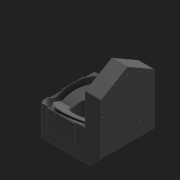
# Autodesk Inventor part: Arm L-Bracket
Saved by Autodesk Inventor 2017 (Build 210142000, 142)
## iProperties
Created: 2019-08-29
Part Number: Arm L-Bracket
Material: ABS Plastic
Document SubType Name: Modeling
Designer: Dell
Density: 1.06 g/cm^3
Appearance: Smooth - Black
Author: Dell
Autodesk Inventor part; units mm, degrees
ref_plane "YZ Plane" through (0, 0, 0) normal (1, 0, 0) x (0, 1, 0)
ref_plane "XZ Plane" through (0, 0, 0) normal (0, 1, 0) x (-1, 0, 0)
ref_plane "XY Plane" through (0, 0, 0) normal (0, 0, 1) x (1, 0, 0)
sketch "Sketch1" plane through (0, 0, 0) normal (0, 0, 1) x (1, 0, 0)
  line L0 (68.1273, 0) -> (34.0637, -59)
  line L1 (34.0637, -59) -> (-34.0637, -59)
  line L2 (-34.0637, -59) -> (-68.1273, 0)
  line L3 (-68.1273, 0) -> (-34.0637, 59)
  line L4 (-34.0637, 59) -> (34.0637, 59)
  line L5 (34.0637, 59) -> (68.1273, 0)
  line L6 (34.0637, 59) -> (43.0281, 59)
  line L7 (43.0281, 59) -> (93.1273, 59)
  line L8 (93.1273, 59) -> (93.1273, -59)
  line L9 (93.1273, -59) -> (34.0637, -59)
  circle A0 centre (0, 0) radius 22.5
  circle A1 centre (-54, 0) radius 2.5
  circle A2 centre (-46.7654, -27) radius 2.5
  circle A3 centre (-27, -46.7654) radius 2.5
  circle A4 centre (0, -54) radius 2.5
  circle A5 centre (27, -46.7654) radius 2.5
  circle A6 centre (46.7654, -27) radius 2.5
  circle A7 centre (54, 0) radius 2.5
  circle A8 centre (46.7654, 27) radius 2.5
  circle A9 centre (27, 46.7654) radius 2.5
  circle A10 centre (0, 54) radius 2.5
  circle A11 centre (-27, 46.7654) radius 2.5
  circle A12 centre (-46.7654, 27) radius 2.5
  dimension "d0" = 118
  dimension "d1" = 25
  dimension "d2" = 45
  dimension "d3" = 54
  dimension "d4" = 5
  dimension "d7" = 360
  constraints: 20 end point, 13 centre point, 2 coincident, 2 horizontal, 2 horizontal alignment, 1 perpendicular, 1 point on line, 38 other
  measures "d0" distance between parallel lines of L1 L4
  measures "d1" distance from line of L8 L0.start
  measures "d2" diameter of A0
  measures "d3" distance of point (0, 0) A1.centre
  measures "d4" diameter of A1
extrude "Extrusion1" add sketch "Sketch1" along normal blind 30
sketch "Sketch2" plane through (93.1273, -59, 0) normal (1, 0, 0) x (0, 0, -1)
  line L0 (-69.0637, 118) -> (-35, 59)
  line L1 (-35, 59) -> (-69.0637, 0)
  line L2 (-69.0637, 0) -> (-137.191, 0)
  line L3 (-137.191, 0) -> (-171.2547, 59)
  line L4 (-171.2547, 59) -> (-137.191, 118)
  line L5 (-137.191, 118) -> (-69.0637, 118)
  line L6 (0, 0) -> (0, 118) projected
  line L7 (0, 0) -> (-69.0637, 0)
  line L8 (0, 118) -> (-30, 118) projected
  line L9 (-69.0637, 118) -> (0, 118)
  line L10 (0, 118) -> (0, 0)
  circle A0 centre (-103.1273, 59) radius 22.5
  circle A1 centre (-157.1273, 59) radius 2.5
  circle A2 centre (-149.8927, 32) radius 2.5
  circle A3 centre (-130.1273, 12.2346) radius 2.5
  circle A4 centre (-103.1273, 5) radius 2.5
  circle A5 centre (-76.1273, 12.2346) radius 2.5
  circle A6 centre (-56.362, 32) radius 2.5
  circle A7 centre (-49.1273, 59) radius 2.5
  circle A8 centre (-56.362, 86) radius 2.5
  circle A9 centre (-76.1273, 105.7654) radius 2.5
  circle A10 centre (-103.1273, 113) radius 2.5
  circle A11 centre (-130.1273, 105.7654) radius 2.5
  circle A12 centre (-149.8927, 86) radius 2.5
  point P0 (0, 59)
  point P1 (-30, 0)
  dimension "d12" = 45
  dimension "d13" = 5
  dimension "d14" = 54
  dimension "d17" = 360
  dimension "d25" = 5
  constraints: 18 end point, 13 centre point, 3 horizontal alignment, 2 perpendicular, 1 coincident, 1 collinear, 1 horizontal, 38 other
  measures "d12" diameter of A0
  measures "d13" diameter of A1
  measures "d14" distance of point (-103.127, 59) A1.centre
  measures "d25" horizontal distance of L8.end L0.end
extrude "Extrusion2" add sketch "Sketch2" against normal blind 30 and the other way blind 5
sketch "Sketch3" plane through (63.1273, -59, 0) normal (-1, 0, 0) x (0, 0, 1)
  circle A0 centre (103.1273, 59) radius 22.5 projected
  line L0 (171.2547, 59) -> (137.191, 0) projected
  line L1 (171.2547, 59) -> (137.191, 0)
  line L2 (137.191, 0) -> (69.0637, 0)
  line L3 (69.0637, 0) -> (35, 59)
  line L4 (35, 59) -> (69.0637, 118)
  line L5 (69.0637, 118) -> (137.191, 118)
  line L6 (137.191, 118) -> (171.2547, 59)
  line L7 (137.191, 118) -> (30, 118) projected
  line L8 (69.0637, 118) -> (30, 118)
  line L9 (30, 0) -> (30, 118) projected
  line L10 (30, 118) -> (30, 0)
  line L11 (30, 0) -> (69.0637, 0)
  point P0 (0, 59)
  constraints: 18 end point, 2 collinear, 1 coincident, 1 perpendicular, 13 other
extrude "Extrusion3" add sketch "Sketch3" along normal blind 180 contours L11 L9 L7 L4 L3
sketch "Sketch4" plane through (0, 0, 0) normal (0, 0, -1) x (-1, 0, 0)
  line L0 (34.0637, -59) -> (-98.1273, -59) projected
  line L1 (68.1273, 0) -> (34.0637, -59) projected
  line L2 (34.0637, 59) -> (68.1273, 0) projected
  line L3 (34.0637, 59) -> (-98.1273, 59) projected
  line L4 (-98.1273, -59) -> (-98.1273, 59) construction
  circle A0 centre (0, 0) radius 22.5 projected
  circle A1 centre (46.7654, 27) radius 2.5 projected
  circle A2 centre (27, 46.7654) radius 2.5 projected
  circle A3 centre (0, 54) radius 2.5 projected
  circle A4 centre (-27, 46.7654) radius 2.5 projected
  circle A5 centre (-46.7654, 27) radius 2.5 projected
  circle A6 centre (-54, 0) radius 2.5 projected
  circle A7 centre (-46.7654, -27) radius 2.5 projected
  circle A8 centre (-27, -46.7654) radius 2.5 projected
  circle A9 centre (0, -54) radius 2.5 projected
  circle A10 centre (27, -46.7654) radius 2.5 projected
  circle A11 centre (46.7654, -27) radius 2.5 projected
  circle A12 centre (54, 0) radius 2.5 projected
  line L5 (34.0637, 59) -> (68.1273, 0) projected
  line L6 (68.1273, 0) -> (34.0637, -59) projected
  line L7 (34.0637, -59) -> (116.8727, -59) projected
  line L8 (116.8727, 59) -> (116.8727, -59) projected
  line L9 (34.0637, 59) -> (116.8727, 59) projected
extrude "Extrusion4" cut sketch "Sketch4" against normal through all
sketch "Sketch5" plane through (98.1273, -59, 0) normal (1, 0, 0) x (0, 0, -1)
  circle A0 centre (-103.1273, 59) radius 22.5 projected
extrude "Extrusion5" add sketch "Sketch5" against normal blind 5
sketch "Sketch6" plane through (63.1273, -59, 0) normal (-1, 0, 0) x (0, 0, 1)
  circle A0 centre (103.1273, 59) radius 22.5 projected
  line L0 (82.8587, 68.7691) -> (46.8217, 79.4757)
  line L1 (80.6273, 59) -> (41.6806, 70.5711)
  line L2 (69.0637, 118) -> (35, 59) projected
  line L3 (69.0637, 118) -> (35, 59) projected
  circle A1 centre (56.362, 86) radius 2.5 construction
  circle A2 centre (49.1273, 59) radius 2.5 construction
  circle A3 centre (56.362, 86) radius 2.5 projected
  line L4 (56.362, 86) -> (54.0392, 77.3314)
  line L5 (49.1273, 59) -> (51.4501, 67.6686)
  line L6 (54.0392, 77.3314) -> (51.4501, 67.6686) construction
  circle A4 centre (49.1273, 59) radius 2.5 projected
  line L7 (103.1273, 59) -> (49.1273, 59) construction
  line L8 (82.8587, 68.7691) -> (80.6273, 59)
  line L9 (46.8217, 79.4757) -> (41.6806, 70.5711)
  point P0 (0, 59)
  dimension "d30" = 10
  constraints: 16 end point, 5 point on line, 4 collinear, 2 point on circle, 1 horizontal, 1 parallel
  measures "d30" distance between parallel lines of L0 L1
extrude "Extrusion6" cut sketch "Sketch6" against normal blind 10 contours L8 A0 | A0 L1 L2 L0 picked at (81.7048, 64.4686)
sketch "Sketch7" plane through (-34.0637, 59, 69.0637) normal (0, -0.5, 0.8660254) x (1, 0, 0)
  ellipse E0 centre (34.0637, -68.1273) end of major axis (34.0637, -42.1466) minor radius 22.5 (56.5637, -68.1273) -> (11.5637, -68.1273) ccw projected
  line L0 (85.5637, -68.1273) -> (56.5637, -68.1273) projected
  ellipse E1 centre (88.0637, -68.1273) end of major axis (88.0637, -65.2406) minor radius 2.5 (90.5637, -68.1273) -> (85.5637, -68.1273) ccw projected
  line L1 (97.191, -68.1273) -> (90.5637, -68.1273) projected
  line L2 (97.191, -54.7661) -> (97.191, -68.1273) projected
  line L3 (97.191, -54.7661) -> (107.191, -54.7661) projected
  line L4 (107.191, -54.7661) -> (107.191, -44.484) projected
  line L5 (97.191, -44.484) -> (107.191, -44.484) projected
  line L6 (97.191, 0) -> (97.191, -44.484) projected
  line L7 (97.191, 0) -> (0, 0) projected
  line L8 (0, 0) -> (-34.0637, -68.1273) projected
  line L9 (-22.4363, -68.1273) -> (-34.0637, -68.1273) projected
  ellipse E2 centre (-19.9363, -68.1273) end of major axis (-19.9363, -65.2406) minor radius 2.5 (-17.4363, -68.1273) -> (-22.4363, -68.1273) ccw projected
  line L10 (11.5637, -68.1273) -> (-17.4363, -68.1273) projected
  ellipse E3 centre (80.829, -36.9504) end of major axis (80.829, -34.0637) minor radius 2.5 projected
  ellipse E4 centre (34.0637, -5.7735) end of major axis (34.0637, -2.8868) minor radius 2.5 projected
  ellipse E5 centre (-12.7017, -36.9504) end of major axis (-12.7017, -34.0637) minor radius 2.5 projected
  ellipse E6 centre (7.0637, -14.1273) end of major axis (7.0637, -11.2406) minor radius 2.5 projected
  ellipse E7 centre (61.0637, -14.1273) end of major axis (61.0637, -11.2406) minor radius 2.5 projected
  line L11 (97.191, -54.7661) -> (56.5637, -68.1273)
  line L12 (88.0637, -68.1273) -> (85.8302, -58.5024)
  line L13 (85.8302, -58.5024) -> (83.6134, -48.9493) construction
  line L14 (83.6134, -48.9493) -> (80.829, -36.9504)
  line L15 (97.191, -44.484) -> (54.9219, -58.3851)
  line L16 (54.9219, -58.3851) -> (56.5637, -68.1273)
  point P0 (34.0637, -85.6273)
  constraints: 12 end point, 3 point on line, 1 collinear, 1 parallel, 9 other
extrude "Extrusion7" cut sketch "Sketch7" against normal blind 10 contours E0 L15 L5 L4 L3 L11
ref_plane "Work Plane1" through (-34.0637, -59, 69.0637) normal (0, 0, -1) x (-1, 0, 0)
chamfer "Chamfer1" distance 25 angle 45 1 edges at (98.1273, 0, 0)
sketch "Sketch9" plane through (63.1273, -59, 0) normal (-1, 0, 0) x (0, 0, 1)
  circle A0 centre (149.8927, 86) radius 2.5 construction
  circle A1 centre (130.1273, 105.7654) radius 2.5 construction
  circle A2 centre (103.1273, 113) radius 2.5 construction
  circle A3 centre (76.1273, 105.7654) radius 2.5 construction
  circle A4 centre (56.362, 86) radius 2.5 construction
  circle A5 centre (49.1273, 59) radius 2.5 construction
  circle A6 centre (56.362, 32) radius 2.5 construction
  circle A7 centre (76.1273, 12.2346) radius 2.5 construction
  circle A8 centre (103.1273, 5) radius 2.5 construction
  circle A9 centre (130.1273, 12.2346) radius 2.5 construction
  circle A10 centre (149.8927, 32) radius 2.5 construction
  circle A11 centre (157.1273, 59) radius 2.5 construction
  line L0 (80.6273, 59) -> (41.6806, 70.5711) construction
  line L1 (41.6806, 70.5711) -> (35, 59) construction
  line L2 (35, 59) -> (69.0637, 0) construction
  line L3 (69.0637, 0) -> (137.191, 0) construction
  line L4 (137.191, 0) -> (171.2547, 59) construction
  line L5 (171.2547, 59) -> (137.191, 118) construction
  line L6 (137.191, 118) -> (69.0637, 118) construction
  line L7 (69.0637, 118) -> (46.8217, 79.4757) construction
  line L8 (46.8217, 79.4757) -> (82.8587, 68.7691) construction
  arc A12 (80.6273, 59) -> (82.8587, 68.7691) centre (103.1273, 59) ccw construction
  line L9 (137.191, 118) -> (171.2547, 59)
  line L10 (171.2547, 59) -> (137.191, 0)
  line L11 (137.191, 0) -> (69.0637, 0)
  line L12 (69.0637, 0) -> (35, 59)
  line L13 (35, 59) -> (69.0637, 118)
  line L14 (69.0637, 118) -> (137.191, 118)
  line L15 (67.909, 120) -> (32.6906, 59)
  line L16 (32.6906, 59) -> (67.909, -2)
  line L17 (67.909, -2) -> (138.3457, -2)
  line L18 (138.3457, -2) -> (173.5641, 59)
  line L19 (173.5641, 59) -> (138.3457, 120)
  line L20 (138.3457, 120) -> (67.909, 120)
  point P0 (0, 59)
  dimension "d44" = 2
  constraints: 24 end point, 1 coincident, 18 other
  measures "d44" distance between parallel lines of L13 L15
extrude "Extrusion9" cut sketch "Sketch9" along normal through all contours L9 L10 L11 L12 L13 L14 | L20 L19 L18 L17 L16 L15
sketch "Sketch11" plane through (-34.0637, 59, 0) normal (-0.8660254, 0.5, 0) x (0, 0, 1)
  line L0 (32.6906, -68.1273) -> (66.7543, 0) projected
  line L1 (40.9724, -51.5637) -> (20, -51.5637)
  line L2 (20, -51.5637) -> (20, -16.5637)
  line L3 (20, -16.5637) -> (58.4724, -16.5637)
  line L4 (58.4724, -16.5637) -> (40.9724, -51.5637)
  line L5 (0, 0) -> (0, -68.1273) projected
  point P0 (0, -34.0637)
  point P1 (20, -34.0637)
  point P2 (0, -34.0637)
  dimension "d49" = 35
  dimension "d50" = 20
  constraints: 8 end point, 2 midpoint, 2 perpendicular, 2 point on line, 1 collinear, 1 horizontal, 1 horizontal alignment
  measures "d49" distance of L1.end L2.end
  measures "d50" distance between parallel lines of L5 L2
extrude "Extrusion11" add sketch "Sketch11" along normal blind 3
mirror "Mirror1" about plane through (0, 0, 0) normal (0, 1, 0) of "Extrusion11"
sketch "Sketch12" plane through (63.1273, 59, 137.191) normal (0, 1, 0) x (1, 0, 0)
  ellipse E0 centre (-63.1273, 73.3235) end of major axis (-60.6273, 73.3235) minor radius 1.4434 projected
  line L0 (-65.6273, 137.191) -> (-60.6273, 137.191) projected
  line L1 (-97.191, 70.4367) -> (0, 70.4367) projected
  line L2 (-80.6273, 70.4367) -> (-80.6273, 117.191)
  line L3 (-80.6273, 117.191) -> (-45.6273, 117.191)
  line L4 (-45.6273, 117.191) -> (-45.6273, 70.4367)
  line L5 (-80.6273, 70.4367) -> (-45.6273, 70.4367)
  line L6 (0, 70.4367) -> (-97.191, 70.4367) projected
  line L7 (-45.6273, 117.191) -> (-20.6273, 117.191)
  line L8 (-20.6273, 117.191) -> (-20.6273, 70.4367)
  line L9 (-20.6273, 70.4367) -> (-45.6273, 70.4367)
  line L10 (-45.6273, 70.4367) -> (-45.6273, 117.191)
  point P0 (-63.1273, 137.191)
  point P1 (-63.1273, 117.191)
  point P2 (-63.1273, 137.191)
  dimension "d56" = 20
  dimension "d57" = 35
  dimension "d60" = 25
  constraints: 16 end point, 4 perpendicular, 3 point on line, 2 midpoint, 2 parallel, 1 horizontal, 1 vertical, 1 vertical alignment, 1 other
  measures "d56" distance between parallel lines of L0 L3
  measures "d57" distance of L2.end L3.end
  measures "d60" distance between parallel lines of L4 L8
extrude "Extrusion12" add sketch "Sketch12" along normal blind 3.5 contours E0 | L2 L3 L4 L1 | L4 L7 L8 L1
mirror "Mirror2" about plane through (0, 0, 0) normal (0, 1, 0) of "Extrusion12"
sketch "Sketch8" plane through (-34.0637, -59, 69.0637) normal (0, 0, -1) x (-1, 0, 0)
  circle A0 centre (-34.0637, 113) radius 2.5 projected
  circle A1 centre (-34.0637, 113) radius 6.5
  circle A2 centre (-34.0637, 59) radius 47.5
  circle A3 centre (-34.0637, 59) radius 22.5 projected
  circle A4 centre (-34.0637, 59) radius 60.5
  dimension "d36" = 13
  constraints: 3 centre point, 3 coincident, 2 tangent
  measures "d36" diameter of A1
extrude "Extrusion8" cut sketch "Sketch8" along normal blind 45 contours A0 | A1 | A4
body "Solid1"
